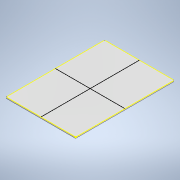
# Autodesk Inventor part: Part1
Saved by Autodesk Inventor 2020.3 (Build 243373000, 373)
## iProperties
Created: 2020-07-15
Part Number: Part1
Material: Generic
Document SubType Name: Modeling
Designer: mifer
Density: 1 g/cm^3
Appearance: Default
Author: mifer
Autodesk Inventor part; units mm, degrees
ref_plane "YZ Plane" through (0, 0, 0) normal (1, 0, 0) x (0, 1, 0)
ref_plane "XZ Plane" through (0, 0, 0) normal (0, 1, 0) x (-1, 0, 0)
ref_plane "XY Plane" through (0, 0, 0) normal (0, 0, 1) x (1, 0, 0)
sketch "Sketch1" plane through (0, 0, 0) normal (0, 1, 0) x (-1, 0, 0)
  line L0 (0, 0) -> (210, 0)
  line L1 (210, 0) -> (210, -297)
  line L2 (210, -297) -> (0, -297)
  line L3 (0, -297) -> (0, 0)
  line L4 (23, -106) -> (187, -106)
  line L5 (187, -106) -> (187, -191)
  line L6 (187, -191) -> (23, -191)
  line L7 (23, -191) -> (23, -106)
  dimension "d30" = 210
  dimension "d31" = 297
  dimension "d34" = 164
  dimension "d35" = 85
  dimension "d42" = 106
  dimension "d43" = 23
  constraints: 16 end point, 4 parallel, 2 horizontal, 2 perpendicular
  measures "d30" distance of L1.end L2.end
  measures "d31" distance of L0.end L1.end
  measures "d34" distance of L5.end L6.end
  measures "d35" distance of L4.end L5.end
  measures "d42" distance between parallel lines of L0 L4
  measures "d43" distance between parallel lines of L7 L3
extrude "Extrusion6" add sketch "Sketch1" against normal blind 4 contours L4 L5 L6 L7
extrude "Extrusion7" add sketch "Sketch1" along normal blind 4 contours L0 L1 L2 L3 | L4 L5 L6 L7
fillet "Fillet3" radius 2 4 edges at (0, 2, 0) (-210, 2, 0) (-210, 2, -297) (0, 2, -297)
fillet "Fillet4" radius 8 4 edges at (-187, -2, -191) (-187, -2, -106) (-23, -2, -106) (-23, -2, -191)
sketch "Sketch3" plane through (0, 4, 0) normal (0, 1, 0) x (1, 0, 0)
  line L0 (-210, 295) -> (-210, 2) projected
  line L1 (-210, 148.5) -> (0, 148.5)
  line L2 (0, 2) -> (0, 295) projected
  line L3 (-208, 0) -> (-2, 0) projected
  line L4 (-105, 0) -> (-105, 297)
  line L5 (-2, 297) -> (-208, 297) projected
  point P0 (0, 0)
  constraints: 4 end point, 4 midpoint
body "Solid3"
